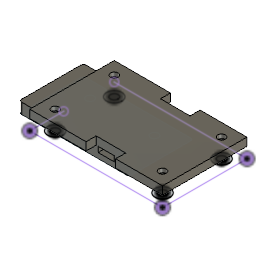
ce51df2b-e6fc-4624-918c-c9696bc77d67 (Autodesk Fusion 360 design; units mm, degrees)
part number: 2026-05-18-20-38-29-636
Autodesk Fusion 360 part; units mm, degrees
note: some values were not read from the file. Set by a fixed rule: which sketch regions a step uses.
sketch "スケッチ1" plane through (0, 0, 0) normal (0, 0, 1) x (1, 0, 0)
  line L0 (0, 0) -> (41, 0)
  line L1 (41, 0) -> (41, 24)
  line L2 (41, 24) -> (0, 24)
  line L3 (0, 24) -> (0, 0)
  dimension "d1" = 24
  dimension "d2" = 41
  constraint horizontal L0
  constraint vertical L1
  constraint horizontal L2
  constraint vertical L3
  constraint coincident L0.start L3.end
  measures "d1" distance of L0.start L2.end
  measures "d2" distance of L0.start L0.end
extrude "押し出し1" add sketch "スケッチ1" along normal blind 4
fillet "フィレット1" radius 1 4 edges at (41, 0, 2) (0, 0, 2) (41, 24, 2) (0, 24, 2)
sketch "スケッチ4" plane through (0, 0, 0) normal (0, 0, -1) x (1, 0, 0)
  arc A0 (0, -23) -> (1, -24) centre (1, -23) ccw
  line L0 (1, -24) -> (40, -24)
  arc A1 (40, -24) -> (41, -23) centre (40, -23) ccw
  line L1 (41, -23) -> (41, -1)
  arc A2 (41, -1) -> (40, 0) centre (40, -1) ccw
  line L2 (40, 0) -> (1, 0)
  arc A3 (1, 0) -> (0, -1) centre (1, -1) ccw
  line L3 (0, -1) -> (0, -23)
  line L4 (8.5, -6) -> (32.5, -6)
  line L5 (32.5, -6) -> (32.5, -18)
  line L6 (32.5, -18) -> (8.5, -18)
  line L7 (8.5, -18) -> (8.5, -6)
  circle A4 centre (8.5, -6) radius 1.45
  circle A5 centre (32.5, -6) radius 1.45
  circle A6 centre (8.5, -18) radius 1.45
  circle A7 centre (32.5, -18) radius 1.45
  dimension "d20" = 24
  dimension "d21" = 12
  dimension "d22" = 41
  dimension "d23" = 8.5
  dimension "d24" = 6
  dimension "d25" = 24
  dimension "d26" = 2.9
  dimension "d27" = 2.9
  dimension "d28" = 2.9
  dimension "d29" = 2.9
  constraint horizontal L4
  constraint vertical L5
  constraint horizontal L6
  constraint vertical L7
  constraint coincident L4.start L7.end
  constraint coincident L4.end L5.start
  constraint coincident L6.end L7.start
  constraint coincident L5.end L6.start
  measures "d20" distance of L4.start L4.end
  measures "d21" distance of L4.start L6.end
  measures "d22" distance of L1 L3
  measures "d23" distance of L3 L7
  measures "d24" distance of L2 L4
  measures "d25" distance of L0 L2
  measures "d26" diameter of A4
  measures "d27" diameter of A5
  measures "d28" diameter of A6
  measures "d29" diameter of A7
extrude "押し出し4" cut sketch "スケッチ4" against normal through all contours L4 L7 A4 | L4 L7 A4 | L4 L5 A5 | L4 L5 A5 | L6 L7 A6 | L6 L7 A6 | L5 L6 A7 | L5 L6 A7
sketch "スケッチ5" plane through (0, 0, 4) normal (0, 0, 1) x (-1, 0, 0)
  circle A0 centre (-8.5, -18) radius 1.45
  circle A1 centre (-8.5, -6) radius 1.45
  line L0 (-40, -24) -> (-1, -24)
  arc A2 (-1, -24) -> (0, -23) centre (-1, -23) ccw
  line L1 (0, -23) -> (0, -1)
  arc A3 (0, -1) -> (-1, 0) centre (-1, -1) ccw
  line L2 (-1, 0) -> (-40, 0)
  circle A4 centre (-8.5, -18) radius 3
  circle A5 centre (-8.5, -6) radius 3
  arc A6 (-40, 0) -> (-41, -1) centre (-40, -1) ccw
  line L3 (-41, -1) -> (-41, -23)
  arc A7 (-41, -23) -> (-40, -24) centre (-40, -23) ccw
  circle A8 centre (-32.5, -18) radius 1.45
  circle A9 centre (-32.5, -6) radius 1.45
  circle A10 centre (-32.5, -18) radius 3
  circle A11 centre (-32.5, -6) radius 3
  dimension "d31" = 6
  dimension "d32" = 6
  dimension "d35" = 6
  dimension "d36" = 6
  constraint concentric A0 A4
  constraint concentric A1 A5
  constraint concentric A8 A10
  constraint concentric A9 A11
  measures "d31" diameter of A4
  measures "d32" diameter of A5
  measures "d35" diameter of A10
  measures "d36" diameter of A11
extrude "押し出し5" cut sketch "スケッチ5" against normal blind 2 contours A4 | A5 | A10 | A11
sketch "スケッチ6" plane through (0, 0, 4) normal (0, 0, 1) x (-1, 0, 0)
  arc A0 (-1, -24) -> (0, -23) centre (-1, -23) ccw
  line L0 (0, -23) -> (0, -1)
  arc A1 (0, -1) -> (-1, 0) centre (-1, -1) ccw
  line L1 (-1, 0) -> (-40, 0)
  arc A2 (-40, 0) -> (-41, -1) centre (-40, -1) ccw
  line L2 (-41, -1) -> (-41, -23)
  arc A3 (-41, -23) -> (-40, -24) centre (-40, -23) ccw
  line L3 (-40, -24) -> (-1, -24)
  circle A4 centre (-32.5, -6) radius 3
  circle A5 centre (-8.5, -18) radius 3
  circle A6 centre (-32.5, -18) radius 3
  circle A7 centre (-8.5, -6) radius 3
  line L4 (-5.5, -6) -> (-11.5, -6)
  line L5 (-11.5, -6) -> (-11.5, 1)
  line L6 (-11.5, 1) -> (-5.5, 1)
  line L7 (-5.5, 1) -> (-5.5, -6)
  line L8 (-5.5, -18) -> (-11.5, -18)
  line L9 (-11.5, -18) -> (-11.5, -25)
  line L10 (-11.5, -25) -> (-5.5, -25)
  line L11 (-5.5, -25) -> (-5.5, -18)
  line L12 (-29.5, -6) -> (-35.5, -6)
  line L13 (-35.5, -6) -> (-35.5, 1)
  line L14 (-35.5, 1) -> (-29.5, 1)
  line L15 (-29.5, 1) -> (-29.5, -6)
  line L16 (-29.5, -18) -> (-35.5, -18)
  line L17 (-35.5, -18) -> (-35.5, -25)
  line L18 (-35.5, -25) -> (-29.5, -25)
  line L19 (-29.5, -25) -> (-29.5, -18)
  dimension "d37" = 6
  dimension "d38" = 7
  dimension "d39" = 6
  dimension "d40" = 7
  dimension "d41" = 6
  dimension "d42" = 7
  dimension "d43" = 6
  dimension "d44" = 7
  constraint horizontal L4
  constraint vertical L5
  constraint horizontal L6
  constraint vertical L7
  constraint coincident A7 L4.start
  constraint horizontal L8
  constraint vertical L9
  constraint horizontal L10
  constraint vertical L11
  constraint coincident A5 L8.start
  constraint horizontal L12
  constraint vertical L13
  constraint horizontal L14
  constraint vertical L15
  constraint coincident A4 L12.start
  constraint horizontal L16
  constraint vertical L17
  constraint horizontal L18
  constraint vertical L19
  constraint coincident A6 L16.start
  measures "d37" distance of L4.start L4.end
  measures "d38" distance of L4.start L6.end
  measures "d39" distance of L8.start L8.end
  measures "d40" distance of L8.start L10.end
  measures "d41" distance of L12.start L12.end
  measures "d42" distance of L12.start L14.end
  measures "d43" distance of L16.start L16.end
  measures "d44" distance of L16.start L18.end
extrude "押し出し6" cut sketch "スケッチ6" against normal blind 2 contours L3 A5 L9 L11 | L3 A6 L17 L19 | L1 A7 L5 L7 | L1 A4 L13 L15
sketch "スケッチ7" plane through (0, 0, 4) normal (0, 0, 1) x (-1, 0, 0)
  line L0 (-35.5, -24) -> (-35.5, -18)
  arc A0 (-29.5, -18) -> (-35.5, -18) centre (-32.5, -18) ccw
  line L1 (-29.5, -18) -> (-29.5, -24)
  line L2 (-29.5, -24) -> (-11.5, -24)
  line L3 (-11.5, -24) -> (-11.5, -18)
  arc A1 (-5.5, -18) -> (-11.5, -18) centre (-8.5, -18) ccw
  line L4 (-5.5, -18) -> (-5.5, -24)
  line L5 (-5.5, -24) -> (-1, -24)
  arc A2 (-1, -24) -> (0, -23) centre (-1, -23) ccw
  line L6 (0, -23) -> (0, -1)
  arc A3 (0, -1) -> (-1, 0) centre (-1, -1) ccw
  line L7 (-1, 0) -> (-5.5, 0)
  line L8 (-5.5, 0) -> (-5.5, -6)
  arc A4 (-11.5, -6) -> (-5.5, -6) centre (-8.5, -6) ccw
  line L9 (-11.5, -6) -> (-11.5, 0)
  line L10 (-11.5, 0) -> (-29.5, 0)
  line L11 (-29.5, 0) -> (-29.5, -6)
  arc A5 (-35.5, -6) -> (-29.5, -6) centre (-32.5, -6) ccw
  line L12 (-35.5, -6) -> (-35.5, 0)
  line L13 (-35.5, 0) -> (-40, 0)
  arc A6 (-40, 0) -> (-41, -1) centre (-40, -1) ccw
  line L14 (-41, -1) -> (-41, -23)
  arc A7 (-41, -23) -> (-40, -24) centre (-40, -23) ccw
  line L15 (-40, -24) -> (-35.5, -24)
  line L16 (-7.75, 3.75) -> (-57.25, 3.75)
  line L17 (-57.25, 3.75) -> (-57.25, -27.75)
  line L18 (-57.25, -27.75) -> (-7.75, -27.75)
  line L19 (-7.75, -27.75) -> (-7.75, 3.75)
  line L20 (-20.5, 3.5024) -> (-20.5, -24.5446)
  dimension "d47" = 49.5
  dimension "d48" = 31.5
  dimension "d49" = 41
  dimension "d50" = 20.5
  dimension "d51" = 12.75
  dimension "d52" = 24
  dimension "d53" = 3.75
  constraint horizontal L16
  constraint vertical L17
  constraint horizontal L18
  constraint vertical L19
  constraint perpendicular L2 L20
  measures "d47" distance of L16.start L16.end
  measures "d48" distance of L16.start L18.end
  measures "d49" distance of L6 L14
  measures "d50" distance of L6 L20
  measures "d51" distance of L19 L20
  measures "d52" distance of L5 L7
  measures "d53" distance of L2 L18
extrude "押し出し7" add sketch "スケッチ7" along normal blind 3 contours L0 A0 L1 L2 L10 L11 A5 L12 L13 A6 L14 A7 L15 L20 | L0 A0 L1 L2 L3 A1 A4 L9 L10 L11 A5 L12 L13 A6 L14 A7 L15 L16 L17 L18 L19 | L2 L3 A1 A4 L9 L10 L19 L20
sketch "スケッチ8" plane through (0, 0, 0) normal (0, 0, -1) x (1, 0, 0)
  circle A0 centre (8.5, -18) radius 1.45
  circle A1 centre (32.5, -6) radius 1.45
  circle A2 centre (8.5, -6) radius 1.45
  circle A3 centre (32.5, -18) radius 1.45
  arc A4 (0, -23) -> (1, -24) centre (1, -23) ccw
  line L0 (1, -24) -> (40, -24)
  arc A5 (40, -24) -> (41, -23) centre (40, -23) ccw
  line L1 (41, -23) -> (41, -1)
  arc A6 (41, -1) -> (40, 0) centre (40, -1) ccw
  line L2 (40, 0) -> (1, 0)
  arc A7 (1, 0) -> (0, -1) centre (1, -1) ccw
  line L3 (0, -1) -> (0, -23)
  line L4 (57.25, 3.75) -> (57.25, -27.75)
  line L5 (7.75, 3.75) -> (57.25, 3.75)
  circle A8 centre (12.5, -1) radius 2.8
  circle A9 centre (12.5, -23) radius 2.8
  circle A10 centre (52.5, -1) radius 2.8
  circle A11 centre (52.5, -23) radius 2.8
  line L6 (57.25, -27.75) -> (7.75, -27.75)
  line L7 (7.75, -8.9047) -> (7.75, 3.75)
  circle A12 centre (12.5, -1) radius 1.4
  circle A13 centre (52.5, -1) radius 1.4
  circle A14 centre (52.5, -23) radius 1.4
  circle A15 centre (12.5, -23) radius 1.4
  dimension "d56" = 31.5
  dimension "d57" = 49.5
  dimension "d58" = 5.6
  dimension "d59" = 5.6
  dimension "d60" = 5.6
  dimension "d61" = 5.6
  dimension "d62" = 40
  dimension "d63" = 40
  dimension "d64" = 40
  dimension "d65" = 22
  dimension "d66" = 22
  dimension "d67" = 22
  dimension "d68" = 4.75
  dimension "d69" = 4.75
  dimension "d72" = 2.8
  dimension "d73" = 2.8
  dimension "d74" = 2.8
  dimension "d75" = 2.8
  constraint concentric A8 A12
  constraint concentric A10 A13
  constraint concentric A11 A14
  constraint concentric A9 A15
  measures "d56" distance of L4.start L4.end
  measures "d57" distance of L4.start L5.start
  measures "d58" diameter of A8
  measures "d59" diameter of A9
  measures "d60" diameter of A10
  measures "d61" diameter of A11
  measures "d62" horizontal distance of A8.centre A10.centre
  measures "d63" horizontal distance of A9.centre A11.centre
  measures "d64" horizontal distance of A8.centre A11.centre
  measures "d65" distance of A10.centre A11.centre
  measures "d66" distance of A8.centre A9.centre
  measures "d67" vertical distance of A8.centre A11.centre
  measures "d68" distance of A9.centre L6
  measures "d69" distance of A8.centre L7
  measures "d72" diameter of A12
  measures "d73" diameter of A13
  measures "d74" diameter of A14
  measures "d75" diameter of A15
extrude "押し出し8" cut sketch "スケッチ8" against normal blind 5.5 contours L0 A9 A15 | L0 A9 A15 | L0 A15 | L0 A15 | L2 A8 A12 | L2 A8 A12 | L2 A12 | L2 A12 | A10 | A11 | A13 | A14
extrude "押し出し9" cut sketch "スケッチ8" against normal through all contours L0 A15 | L0 A15 | L2 A12 | L2 A12 | A13 | A14
sketch "スケッチ9" plane through (0, 0, 7) normal (0, 0, 1) x (-1, 0, 0)
  circle A0 centre (-12.5, -23) radius 1.4
  circle A1 centre (-52.5, -23) radius 1.4
  circle A2 centre (-12.5, -1) radius 1.4
  circle A3 centre (-52.5, -1) radius 1.4
  line L0 (-7.75, -27.75) -> (-7.75, 3.75)
  line L1 (-7.75, 3.75) -> (-57.25, 3.75)
  line L2 (-57.25, 3.75) -> (-57.25, -27.75)
  line L3 (-57.25, -27.75) -> (-7.75, -27.75)
  line L4 (-60, 0) -> (3, 0)
  line L5 (-60, -24) -> (3, -24)
  line L6 (-39.75, -24) -> (-28.75, -24)
  line L7 (-28.75, -24) -> (-28.75, -27.75)
  line L8 (-28.75, -27.75) -> (-39.75, -27.75)
  line L9 (-39.75, -27.75) -> (-39.75, -24)
  line L10 (-39.75, 0) -> (-28.75, 0)
  line L11 (-28.75, 0) -> (-28.75, 3.75)
  line L12 (-28.75, 3.75) -> (-39.75, 3.75)
  line L13 (-39.75, 3.75) -> (-39.75, 0)
  dimension "d77" = 21
  dimension "d78" = 21
  dimension "d79" = 11
  dimension "d80" = 11
  constraint perpendicular L0 L4
  constraint perpendicular L0 L5
  constraint horizontal L6
  constraint vertical L7
  constraint horizontal L8
  constraint vertical L9
  constraint coincident L3 L7.end
  constraint coincident L5 L6.start
  constraint horizontal L10
  constraint vertical L11
  constraint horizontal L12
  constraint vertical L13
  constraint coincident L1 L11.end
  constraint coincident L4 L10.start
  measures "d77" distance of L0 L11
  measures "d78" distance of L0 L7
  measures "d79" distance of L7 L9
  measures "d80" distance of L11 L13
extrude "押し出し10" cut sketch "スケッチ9" against normal through all contours L3 L5 L6 L7 L8 L9 | L1 L4 L10 L11 L12 L13
equation "d23 = ( d22 - d20 ) / 2"
equation "d24 = ( d25 - d21 ) / 2"
equation "d50 = d49 / 2"
equation "d53 = ( d48 - d52 ) / 2"
equation "d59 = d58"
equation "d60 = d58"
equation "d61 = d58"
equation "d68 = ( d56 - d67 ) / 2"
equation "d69 = ( d57 - d64 ) / 2"
